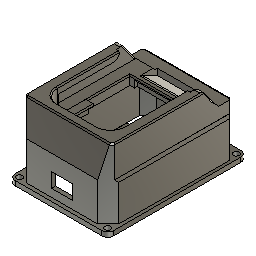
Makita_DIY_Akkulampe (Autodesk Fusion 360 design; units mm, degrees)
Autodesk Fusion 360 part; units mm, degrees
note: some values were not read from the file. Chosen so that the rebuilt part matches the saved one: a side; which face or edge a step refers to; which pieces of a blend or face edit are solid. Set by a fixed rule: which sketch regions a step uses.
sketch "Sketch1" plane through (0, 0, 0) normal (0, 0, 1) x (1, 0, 0)
  line L0 (42.5, 60) -> (-42.5, 60)
  line L1 (-42.5, 60) -> (-42.5, -60)
  line L2 (-42.5, -60) -> (42.5, -60)
  line L3 (42.5, -60) -> (42.5, 60)
  line L4 (42.5, 60) -> (-42.5, -60) construction
  line L5 (-42.5, 60) -> (42.5, -60) construction
  line L6 (-38, 55.5) -> (38, 55.5) construction
  line L7 (38, 55.5) -> (38, -55.5) construction
  line L8 (38, -55.5) -> (-38, -55.5) construction
  line L9 (-38, -55.5) -> (-38, 55.5) construction
  line L10 (-38, 55.5) -> (38, -55.5) construction
  line L11 (38, 55.5) -> (-38, -55.5) construction
  circle A0 centre (-38, -55.5) radius 2.5
  circle A1 centre (38, -55.5) radius 2.5
  circle A2 centre (38, 55.5) radius 2.5
  circle A3 centre (-38, 55.5) radius 2.5
  line L12 (29.2374, -53.4062) -> (-29.365, -53.4062)
  line L13 (-29.365, 53.5938) -> (29.4929, 53.5938)
  line L14 (36.3085, -53.4062) -> (-36.436, 53.5938) construction
  line L15 (-36.436, -53.4062) -> (36.564, 53.5938) construction
  line L16 (-36.436, -46.3352) -> (-29.365, -53.4062)
  line L17 (29.2374, -53.4062) -> (36.3085, -46.3352)
  line L18 (29.4929, 53.5938) -> (36.564, 46.5227)
  line L19 (-36.436, 46.5227) -> (-29.365, 53.5938)
  line L20 (-32.9005, 50.0582) -> (-36.436, 53.5938) construction
  line L21 (33.0284, 50.0582) -> (36.564, 53.5938) construction
  line L22 (32.773, -49.8707) -> (36.3085, -53.4062) construction
  line L23 (-36.436, -53.4062) -> (-32.9005, -49.8707) construction
  line L24 (-36.436, -46.3352) -> (-36.436, 46.5227)
  line L25 (36.564, 46.5227) -> (36.3085, -46.3352)
  line L26 (-29.862, 54.7938) -> (29.99, 54.7938)
  line L27 (29.99, 54.7938) -> (37.7653, 47.0184)
  line L28 (37.7653, 47.0184) -> (37.5071, -46.8336)
  line L29 (29.7345, -54.6062) -> (37.5071, -46.8336)
  line L30 (29.7345, -54.6062) -> (-29.862, -54.6062)
  line L31 (-37.636, -46.8322) -> (-29.862, -54.6062)
  line L32 (-37.636, -46.8322) -> (-37.636, 47.0198)
  line L33 (-37.636, 47.0198) -> (-29.862, 54.7938)
  line L34 (-30.8147, 57.0938) -> (30.9427, 57.0938)
  line L35 (30.9427, 57.0938) -> (40.068, 47.9685)
  line L36 (40.068, 47.9685) -> (39.8045, -47.7889)
  line L37 (30.6872, -56.9062) -> (39.8045, -47.7889)
  line L38 (30.6872, -56.9062) -> (-30.8147, -56.9062)
  line L39 (-39.936, -47.7849) -> (-30.8147, -56.9062)
  line L40 (-39.936, -47.7849) -> (-39.936, 47.9725)
  line L41 (-39.936, 47.9725) -> (-30.8147, 57.0938)
  line L42 (31.5, -44.5) -> (-31.5, 44.5) construction
  line L43 (-31.5, -44.5) -> (31.5, 44.5) construction
  line L44 (-28.5365, 51.5938) -> (28.6645, 51.5938)
  line L45 (28.6645, 51.5938) -> (34.5617, 45.6966)
  line L46 (34.5617, 45.6966) -> (34.3108, -45.5044)
  line L47 (28.409, -51.4062) -> (34.3108, -45.5044)
  line L48 (28.409, -51.4062) -> (-28.5365, -51.4062)
  line L49 (-34.436, -45.5067) -> (-28.5365, -51.4062)
  line L50 (-34.436, -45.5067) -> (-34.436, 45.6943)
  line L51 (-34.436, 45.6943) -> (-28.5365, 51.5938)
  dimension "d1" = 85
  dimension "d2" = 120
  dimension "d3" = 76
  dimension "d4" = 111
  dimension "d5" = 5
  dimension "d6" = 73
  dimension "d7" = 107
  dimension "d9" = 10
  dimension "d10" = 1.2
  dimension "d11" = 3.5
  dimension "d20" = 89
  dimension "d21" = 63
  dimension "d33" = 2
  constraint perpendicular L0 L1
  constraint parallel L0 L2
  constraint parallel L1 L3
  constraint horizontal L0
  constraint perpendicular L6 L7
  constraint parallel L6 L8
  constraint parallel L7 L9
  constraint horizontal L6
  constraint coincident L8.end L9.start
  constraint coincident L7.end L8.start
  constraint coincident L6.end L7.start
  constraint coincident L6.start L9.end
  constraint equal A0 A1
  constraint equal A0 A3
  constraint equal A2 A3
  constraint perpendicular L12 L24
  constraint parallel L12 L13
  constraint horizontal L12
  constraint midpoint L19 L20.start
  constraint perpendicular L19 L20
  constraint midpoint L18 L21.start
  constraint perpendicular L18 L21
  constraint midpoint L17 L22.start
  constraint perpendicular L17 L22
  constraint midpoint L16 L23.end
  constraint perpendicular L16 L23
  constraint equal L22 L23
  constraint equal L20 L23
  constraint equal L20 L21
  constraint horizontal L15.start L12.end
  constraint vertical L15.start L16.start
  constraint vertical L14.start L17.end
  constraint horizontal L14.start L12.start
  constraint horizontal L15.end L13.end
  constraint vertical L15.end L18.end
  constraint vertical L14.end L19.start
  constraint horizontal L14.end L13.start
  measures "d1" distance of L1.end L2.end
  measures "d2" distance of L0.end L1.end
  measures "d3" distance of L7.end L8.end
  measures "d4" distance of L6.end L7.end
  measures "d5" diameter of A2
  measures "d6" distance of L14.end L15.end
  measures "d7" distance of L15.start L14.end
  measures "d9" distance of L13.end L18.end
  measures "d20" distance of L42.start L43.end
  measures "d21" distance of L42.start L43.start
extrude "Extrude5" add sketch "Sketch1" against normal blind 2 contours L0 L1 L2 L3 | L12 L13 L16 L17 L18 L19 L24 L25 | L26 L27 L28 L29 L30 L31 L32 L33 | L44 L45 L46 L47 L48 L49 L50 L51 makes body 1 at (10.2291, -58.9687, 0) makes body 2 at (12.5455, 15.7349, 0)
extrude "Extrude6" add sketch "Sketch1" along normal blind 2 contours L0 L1 L2 L3 | L12 L13 L16 L17 L18 L19 L24 L25 | L26 L27 L28 L29 L30 L31 L32 L33 | L34 L35 L36 L37 L38 L39 L40 L41 | L44 L45 L46 L47 L48 L49 L50 L51 bodies 1 2
sketch "Sketch1 (2)" plane through (0, 0, 0) normal (0, 0, 1) x (1, 0, 0) in component "Contacts"
  line L0 (0, 21.9) -> (8.9, 21.9)
  line L1 (8.9, 21.9) -> (8.9, -21.9)
  line L2 (8.9, -21.9) -> (0, -21.9)
  line L3 (8.9, 14.4) -> (24.3, 14.4)
  line L4 (24.3, 14.4) -> (24.3, -14.4)
  line L5 (24.3, -14.4) -> (8.9, -14.4)
  line L6 (0, 21.9) -> (-30.1, 21.9)
  line L7 (-30.1, 21.9) -> (-30.1, -21.9)
  line L8 (-30.1, -21.9) -> (0, -21.9)
  line L9 (0, -21.9) -> (0, 21.9)
  line L10 (8.9, 14.4) -> (26.7, 14.4)
  line L11 (26.7, 14.4) -> (26.7, 18.8)
  line L12 (26.7, 18.8) -> (8.9, 18.8)
  line L13 (8.9, 18.8) -> (8.9, 14.4)
  line L14 (8.9, -14.4) -> (26.7, -14.4)
  line L15 (26.7, -14.4) -> (26.7, -18.8)
  line L16 (26.7, -18.8) -> (8.9, -18.8)
  line L17 (8.9, -18.8) -> (8.9, -14.4)
  line L18 (-30.1, 17.6) -> (0, 17.6)
  line L19 (0, -17.6) -> (-30.1, -17.6)
  line L20 (-30.1, -17.6) -> (-30.1, 17.6)
  line L21 (-30.1, 17.6) -> (-32.5, 17.6)
  line L22 (-32.5, 17.6) -> (-32.5, -17.6)
  line L23 (-32.5, -17.6) -> (-30.1, -17.6)
  line L24 (-30.1, -17.6) -> (-30.1, 17.6)
  line L25 (0, 0) -> (41.4806, 0) construction
  point P0 (24.3, 0)
  dimension "d34" = 28.8
  dimension "d35" = 15.4
  dimension "d36" = 17.8
  dimension "d39" = 54.4
  dimension "d40" = 24.3
  dimension "d41" = 4.3
  dimension "d42" = 2.4
  dimension "d43" = 35.2
  dimension "d44" = 37.6
  constraint horizontal L0
  constraint vertical L1
  constraint horizontal L2
  constraint horizontal L3
  constraint vertical L4
  constraint horizontal L5
  constraint coincident L1 L3.start
  constraint horizontal L6
  constraint vertical L7
  constraint horizontal L8
  constraint vertical L9
  constraint horizontal L10
  constraint vertical L11
  constraint horizontal L12
  constraint vertical L13
  constraint horizontal L14
  constraint vertical L15
  constraint horizontal L16
  constraint vertical L17
  constraint collinear L11 L15
  constraint equal L11 L15
  constraint horizontal L18
  constraint horizontal L19
  constraint vertical L20
  constraint coincident L7 L18.start
  constraint midpoint L7 L20
  constraint horizontal L21
  constraint vertical L22
  constraint horizontal L23
  constraint vertical L24
  constraint coincident L19.end L20.start
  constraint midpoint L25.start L9
  constraint coincident L1 L5.end
  constraint coincident L25.start origin
  constraint coincident L4 P0
  constraint midpoint L4 P0
  constraint coincident L25 P0
  constraint coincident L9 L18.end
  constraint coincident L9 L19.start
  constraint coincident L2.end L8.end
  constraint horizontal L25
  measures "d34" distance of L3.start L5.end
  measures "d35" distance of L3.start L3.end
  measures "d36" distance of L11.end L12.end
  measures "d39" distance of L4 L7
  measures "d40" horizontal distance of L0.start L3.end
  measures "d41" distance of L6.end L18.start
  measures "d42" distance of L22.end L19.end
  measures "d43" distance of L18.start L19.end
  measures "d44" distance of L11.end L15.end
extrude "Extrude1" add sketch "Sketch1 (2)" along normal blind 2 separate body contours L7 L9 L18 L19 L20 L24 | L1 L3 L10 L11 L12 L13 | L1 L5 L14 L15 L16 L17 makes body 3 at (-20.0667, 5.8667, 0) makes body 4 at (14.8333, -17.3333, 0) makes body 5 at (14.8333, 15.8667, 0) in component "Contacts"
extrude "Extrude2" add sketch "Sketch1 (2)" along normal blind 13.5 contours L0 L1 L2 L9 L13 L17 | L1 L3 L4 L5 L10 L14 bodies 3 4 5 in component "Contacts"
extrude "Extrude3" add sketch "Sketch1 (2)" along normal blind 4.5 contours L6 L7 L9 L18 | L7 L8 L9 L19 bodies 3 in component "Contacts"
extrude "Extrude4" add sketch "Sketch1 (2)" against normal blind 2 separate body contours L7 L20 L21 L22 L23 L24 makes body 6 in component "Contacts"
extrude "Extrude5'" add 1 faces at (-30.1, 5.8667, -0.6667) along direction (1, 0, 0) blind 2 on bodies 6 bodies 6 3 in component "Contacts"
sketch "Sketch2" plane through (0, 0, 4.5) normal (0, 0, 1) x (-1, 0, 0) in component "Contacts"
  line L0 (30.1, -17.6) -> (0, -17.6)
  line L1 (0, -17.6) -> (0, -21.9)
  line L2 (0, -21.9) -> (30.1, -21.9)
  line L3 (30.1, -21.9) -> (30.1, -17.6)
  line L4 (25.4, -20) -> (0, -20)
  line L5 (0, -20) -> (0, -19)
  line L6 (0, -19) -> (25.4, -19)
  line L7 (25.4, -19) -> (25.4, -20)
  line L8 (25.4, 19) -> (0, 19)
  line L9 (0, 19) -> (0, 20)
  line L10 (0, 20) -> (25.4, 20)
  line L11 (25.4, 20) -> (25.4, 19)
  line L12 (0, 0) -> (12.7, 0) construction
  line L13 (12.7, 0) -> (12.7, -19) construction
  line L14 (12.7, 0) -> (12.7, 19) construction
  dimension "d55" = 40
  dimension "d56" = 1
  dimension "d57" = 25.4
  constraint horizontal L4
  constraint vertical L5
  constraint horizontal L6
  constraint vertical L7
  constraint coincident L1 L5.end
  constraint horizontal L8
  constraint vertical L9
  constraint horizontal L10
  constraint vertical L11
  constraint collinear L7 L11
  constraint coincident L12.start origin
  constraint parallel L6 L12
  constraint midpoint L6 L13.end
  constraint perpendicular L6 L13
  constraint midpoint L8 L14.end
  constraint perpendicular L8 L14
  constraint equal L13 L14
  constraint equal L7 L11
  measures "d55" distance of L4.start L10.end
  measures "d56" distance of L4.start L6.end
  measures "d57" distance of L5.end L6.end
extrude "Extrude6'" add sketch "Sketch2" along normal blind 8.3 contours L1 L4 L5 L6 L7 | L8 L9 L10 L11 bodies 6 in component "Contacts"
extrude "Extrude7" add sketch "Sketch1" along normal blind 35 contours L26 L27 L28 L29 L30 L31 L32 L33 | L34 L35 L36 L37 L38 L39 L40 L41 bodies 1
extrude "Extrude8" cut 1 faces at (12.1455, 15.5701, 2) along direction (0, 0, -1) blind 26 on bodies 1 bodies 1
sketch "Sketch2 (2)" plane through (0, 0, 35) normal (0, 0, 1) x (-1, 0, 0)
  line L0 (29.365, 53.4062) -> (36.436, 46.3352)
  line L1 (36.436, 46.3352) -> (36.436, -46.5227)
  line L2 (36.436, -46.5227) -> (29.365, -53.5938)
  line L3 (29.365, -53.5938) -> (-29.4929, -53.5938)
  line L4 (-29.4929, -53.5938) -> (-36.564, -46.5227)
  line L5 (-36.564, -46.5227) -> (-36.3085, 46.3352)
  line L6 (-36.3085, 46.3352) -> (-29.2374, 53.4062)
  line L7 (-29.2374, 53.4062) -> (29.365, 53.4062)
  line L8 (39.936, 47.7849) -> (30.8147, 56.9062)
  line L9 (30.8147, 56.9062) -> (-30.6872, 56.9062)
  line L10 (-30.6872, 56.9062) -> (-39.8045, 47.7889)
  line L11 (-39.8045, 47.7889) -> (-40.068, -47.9685)
  line L12 (-40.068, -47.9685) -> (-30.9427, -57.0938)
  line L13 (-30.9427, -57.0938) -> (30.8147, -57.0938)
  line L14 (30.8147, -57.0938) -> (39.936, -47.9725)
  line L15 (39.936, -47.9725) -> (39.936, 47.7849)
  line L16 (-38, -51.65) -> (38, -51.65)
  line L17 (38, -51.65) -> (38, 51.65)
  line L18 (38, 51.65) -> (-38, 51.65)
  line L19 (-38, 51.65) -> (-38, -51.65)
  line L20 (-38, -51.65) -> (38, 51.65) construction
  line L21 (38, -51.65) -> (-38, 51.65) construction
  line L22 (29, -38.65) -> (29, 32.03)
  line L23 (-29, 32.03) -> (-29, -38.65)
  line L24 (17, 44.03) -> (-17, 44.03)
  arc A0 (29, 32.03) -> (17, 44.03) centre (17, 32.03) ccw
  arc A1 (-17, 44.03) -> (-29, 32.03) centre (-17, 32.03) ccw
  line L25 (38, -38.65) -> (-38, -38.65)
  line L26 (-17, -28.3) -> (17, -28.3)
  line L27 (17, -28.3) -> (17, -42.3)
  line L28 (17, -42.3) -> (-17, -42.3)
  line L29 (-17, -42.3) -> (-17, -28.3)
  line L30 (-17, -28.3) -> (17, -42.3) construction
  line L31 (17, -28.3) -> (-17, -42.3) construction
  line L32 (0, -35.3) -> (0, -51.65) construction
  line L33 (-22, -23.65) -> (22, -23.65)
  line L34 (22, -23.65) -> (22, 15.55)
  line L35 (22, 15.55) -> (-22, 15.55)
  line L36 (-22, 15.55) -> (-22, -23.65)
  line L37 (-22, -23.65) -> (22, 15.55) construction
  line L38 (22, -23.65) -> (-22, 15.55) construction
  line L39 (14.5, 15.55) -> (-14.5, 15.55)
  line L40 (-14.5, 15.55) -> (-14.5, 30.65)
  line L41 (-14.5, 30.65) -> (14.5, 30.65)
  line L42 (14.5, 30.65) -> (14.5, 15.55)
  point P0 (0, -35.3)
  point P1 (0, -4.05)
  dimension "d64" = 76
  dimension "d65" = 103.3
  dimension "d66" = 7.62
  dimension "d67" = 9
  dimension "d68" = 9
  dimension "d69" = 12
  dimension "d70" = 12
  dimension "d71" = 13
  dimension "d72" = 9.35
  dimension "d73" = 34
  dimension "d74" = 14
  dimension "d76" = 28
  dimension "d77" = 44
  dimension "d78" = 39.2
  dimension "d79" = 54.3
  dimension "d80" = 29
  constraint perpendicular L16 L17
  constraint parallel L16 L18
  constraint parallel L17 L19
  constraint horizontal L16
  constraint coincident L20 origin
  constraint coincident L21 origin
  constraint vertical L22
  constraint parallel L22 L23
  constraint perpendicular L22 L24
  constraint tangent L22 A0
  constraint tangent L24 A0
  constraint tangent L24 A1
  constraint tangent L23 A1
  constraint coincident L17 L25.start
  constraint coincident L19 L25.end
  constraint perpendicular L19 L25
  constraint perpendicular L26 L27
  constraint parallel L26 L28
  constraint parallel L27 L29
  constraint horizontal L26
  constraint coincident L30 P0
  constraint coincident L31 P0
  constraint midpoint L31 P0
  constraint coincident P0 L32.start
  constraint midpoint L16 L32.end
  constraint vertical L32
  constraint horizontal L22.start L23.end
  constraint coincident L22.start L25
  constraint perpendicular L33 L34
  constraint parallel L33 L35
  constraint parallel L34 L36
  constraint horizontal L33
  constraint coincident L37 P1
  constraint coincident L38 P1
  constraint vertical origin P1
  constraint horizontal L39
  constraint vertical L40
  constraint horizontal L41
  constraint vertical L42
  constraint coincident L35 L39.start
  constraint midpoint L35 L39
  measures "d64" distance of L16.start L16.end
  measures "d65" distance of L16.start L18.end
  measures "d66" distance of L18 L24
  measures "d67" distance of L17 L22
  measures "d68" distance of L19 L23
  measures "d69" radius of A0
  measures "d70" radius of A1
  measures "d71" distance of L16 L25
  measures "d72" distance of L16 L28
  measures "d73" distance of L27.end L28.end
  measures "d74" distance of L26.start L28.end
  measures "d76" distance of L16 L33
  measures "d77" distance of L34.end L35.end
  measures "d78" distance of L33.end L34.end
  measures "d79" distance of L33 L40.end
  measures "d80" distance of L40.end L41.end
extrude "Extrude9" add sketch "Sketch2 (2)" along normal blind 27 contours L0 L1 L8 L17 L18 L25 | L0 L1 L5 L6 L18 L22 L23 L24 A0 A1 L25 | L5 L6 L10 L18 L19 L25 bodies 1
extrude "Extrude10" add sketch "Sketch2 (2)" along normal blind 11.8 contours L22 L23 L24 A0 A1 L25 L26 L27 L29 bodies 1
extrude "Extrude11" add sketch "Sketch2 (2)" along normal blind 10.1 separate body contours L1 L2 L14 L16 L17 L25 | L1 L2 L4 L5 L16 L25 L27 L28 L29 | L4 L5 L12 L16 L19 L25 makes body 7
sketch "Sketch3" plane through (0, 0, 0) normal (1, 0, 0) x (0, 1, 0)
  line L0 (38.65, 46.8) -> (-32.03, 46.8)
  line L1 (-51.65, 35) -> (-51.65, 62)
  line L2 (-51.65, 62) -> (-51.65, 35)
  line L3 (-35.598, 46.8) -> (31.1855, 46.8)
  line L4 (31.1855, 46.8) -> (31.1855, 56.4)
  line L5 (31.1855, 56.4) -> (-31.35, 56.4)
  line L6 (31.1855, 56.4) -> (21.65, 56.4)
  line L7 (21.65, 56.4) -> (21.65, 62)
  line L8 (21.65, 62) -> (31.1855, 62)
  line L9 (31.1855, 62) -> (31.1855, 56.4)
  line L10 (-31.35, 56.4) -> (-31.35, 46.8)
  line L11 (38.65, 62) -> (-32.03, 62)
  line L12 (38.65, 46.8) -> (27.65, 62)
  line L13 (38.65, 62) -> (38.65, 46.8)
  line L14 (42.3, 35) -> (42.3, 45.1)
  line L15 (42.3, 45.1) -> (42.3, 35)
  line L16 (28.3, 35) -> (28.3, 46.8)
  line L17 (28.3, 46.8) -> (28.3, 35)
  line L18 (42.3, 35) -> (28.3, 35)
  line L19 (28.3, 46.8) -> (42.3, 39.6)
  dimension "d87" = 20.3
  dimension "d88" = 73.3
  dimension "d89" = 5.6
  dimension "d90" = 79.3
  dimension "d95" = 5.5
  constraint horizontal L3
  constraint vertical L4
  constraint horizontal L5
  constraint horizontal L6
  constraint vertical L7
  constraint horizontal L8
  constraint vertical L9
  constraint perpendicular L0 L10
  constraint horizontal L8.end L11.start
  constraint coincident L3 L10.end
  constraint coincident L0.end L3
  constraint coincident L0.start L12.start
  constraint coincident L11 L12.end
  constraint coincident L11.start L13.start
  constraint coincident L14.start L15.end
  constraint coincident L16.start L17.end
  constraint coincident L16.end L17.start
  constraint coincident L15 L19.end
  measures "d87" distance of L2 L5.end
  measures "d88" distance of L1.end L7
  measures "d89" vertical distance of L5.end L11.end
  measures "d90" distance of L1.end L12.end
  measures "d95" distance of L14.end L19.end
extrude "Extrude12" cut sketch "Sketch3" along normal up to surface (38 mm away) contours L9 L11 L12 L13 | L8 L9 L11 L12 bodies 1
extrude "Extrude13" cut sketch "Sketch3" along normal up to surface (31.9 mm away) contours L0 L4 L9 L12 | L0 L3 L4 L5 L6 L10 | L5 L6 L7 L8 L9 L11 L12 bodies 1
extrude "Extrude14" add sketch "Sketch3" along normal up to surface (17 mm away) contours L14 L15 L16 L17 L18 L19 bodies 1 7
mirror "Mirror1" about plane through (0, 0, 0) normal (1, 0, 0) of "Extrude12", "Extrude13", "Extrude14"
sketch "Sketch4" plane through (0, 0, 35) normal (0, 0, 1) x (1, 0, 0)
  line L0 (22, 23.65) -> (-22, 23.65)
  line L1 (18, 23.65) -> (-18, 23.65)
  line L2 (-18, 23.65) -> (-18, 26.15)
  line L3 (-18, 26.15) -> (18, 26.15)
  line L4 (18, 26.15) -> (18, 23.65)
  line L5 (0, 0) -> (0, 23.65) construction
  line L6 (-14.5, -15.55) -> (14.5, -15.55)
  line L7 (-18.9, -15.55) -> (18.9, -15.55)
  line L8 (18.9, -15.55) -> (18.9, -33.05)
  line L9 (18.9, -33.05) -> (-18.9, -33.05)
  line L10 (-18.9, -33.05) -> (-18.9, -15.55)
  line L11 (-22, -15.55) -> (22, -15.55)
  line L12 (14.5, -15.55) -> (14.5, -30.65)
  line L13 (14.5, -30.65) -> (-14.5, -30.65)
  line L14 (-14.5, -30.65) -> (-14.5, -15.55)
  line L15 (-20.9, -13.55) -> (20.9, -13.55)
  line L16 (20.9, -13.55) -> (20.9, -35.05)
  line L17 (20.9, -35.05) -> (-20.9, -35.05)
  line L18 (-20.9, -35.05) -> (-20.9, -13.55)
  line L19 (17, -44.03) -> (-17, -44.03)
  line L20 (-14.5, -30.65) -> (-14.5, -33.05)
  line L21 (14.5, -30.65) -> (14.5, -33.05)
  line L22 (-14.5, -33.05) -> (-14.5, -44.03)
  line L23 (14.5, -33.05) -> (14.5, -44.03)
  dimension "d99" = 36
  dimension "d100" = 2.5
  dimension "d103" = 37.8
  dimension "d104" = 17.5
  dimension "d110" = -2
  constraint horizontal L1
  constraint vertical L2
  constraint horizontal L3
  constraint vertical L4
  constraint coincident L0 L1.start
  constraint coincident L5.start origin
  constraint midpoint L1 L5.end
  constraint vertical L5
  constraint horizontal L7
  constraint vertical L8
  constraint horizontal L9
  constraint vertical L10
  constraint midpoint L7 L11
  constraint coincident L13.end L14.start
  constraint coincident L9 L20.end
  constraint perpendicular L9 L20
  constraint coincident L12.end L13.start
  constraint coincident L9 L21.end
  constraint perpendicular L9 L21
  constraint coincident L19 L22.end
  constraint perpendicular L19 L22
  constraint coincident L19 L23.end
  constraint perpendicular L19 L23
  measures "d99" distance of L2.end L3.end
  measures "d100" distance of L1.end L2.end
  measures "d103" distance of L8.end L9.end
  measures "d104" distance of L7.end L8.end
extrude "Extrude15" cut sketch "Sketch4" along normal up to surface (9.8 mm away) contours L0 L1 L2 L3 L4 bodies 1
extrude "Extrude16" cut sketch "Sketch4" along normal up to surface (11.8 mm away) contours L7 L9 L10 L11 L14 L20 | L6 L7 L11 L12 L13 L14 | L7 L8 L9 L11 L12 L21 | L9 L13 L20 L21 | L9 L17 L22 L23 | L17 L19 L22 L23 bodies 1
extrude "Extrude17" add sketch "Sketch4" along normal blind 2 from surface at 11.8 contours L7 L9 L10 L11 L14 L20 | L7 L8 L9 L11 L12 L21 | L9 L10 L11 L17 L18 L22 | L8 L9 L11 L16 L17 L23 bodies 1
sketch "Sketch5" plane through (0, 0, 0) normal (1, 0, 0) x (0, 1, 0)
  line L0 (-51.65, 35) -> (-51.65, 62)
  line L1 (-51.65, 62) -> (-51.65, 35)
  line L2 (-51.65, 35) -> (-53.4062, 35)
  line L3 (-53.4062, 35) -> (-51.65, 35)
  line L4 (-51.65, 35) -> (-56.9062, 35)
  line L5 (-56.9062, 35) -> (-51.65, 35)
  line L6 (-56.9062, 35) -> (-51.65, 62)
  line L7 (51.65, 35) -> (53.5938, 35)
  line L8 (53.5938, 35) -> (51.65, 35)
  line L9 (51.65, 35) -> (57.0938, 35)
  line L10 (57.0938, 35) -> (51.65, 35)
  line L11 (51.65, 35) -> (51.65, 45.1)
  line L12 (51.65, 45.1) -> (51.65, 35)
  line L13 (57.0938, 35) -> (51.65, 45.1)
  constraint coincident L4.end L5.start
  constraint coincident L0.end L1.start
  constraint coincident L9.end L10.start
  constraint coincident L11.end L12.start
extrude "Extrude18" add sketch "Sketch5" along normal mid plane 74 bodies 1
extrude "Extrude19" cut 4 faces at (34.5435, -55.1541, 35) (34.7764, 55.2792, 35) (-34.6911, 55.2792, 35) (-34.6285, -55.1541, 35) along direction (0, 0, 1) blind 37 on bodies 1 bodies 1
chamfer "Chamfer4" distance 1.7 angle 45 2 edges at (27.5, 38.65, 45.1) (-27.5, 38.65, 45.1) on bodies 1
fillet "Fillet2" radius 1 2 edges at (-20.9, -25.3, 46.8) (20.9, -25.3, 46.8) on bodies 1
fillet "Fillet3" radius 5 8 edges at (34.95, 27.65, 62) (-34.95, 27.65, 62) (30.45, 21.65, 56.4) (-30.45, 21.65, 56.4) (42.5, 60, 0) (-42.5, 60, 0) (42.5, -60, 0) (-42.5, -60, 0) on bodies 1
chamfer "Chamfer5" distance 1 angle 45 21 edges at (-38, -11.0355, 62) (-37.0355, -50.6855, 62) (-0.0638, -51.65, 62) (38, -10.9717, 62) (36.9717, -50.6217, 62) (0, 23.65, 46.8) (22, 4.05, 46.8) (14.5, -39.54, 46.8) (-14.5, -39.54, 46.8) (-22, 4.05, 46.8) (0.064, 51.65, 45.1) (29, -5.19, 62) (25.4853, -40.5153, 62) (0, -44.03, 62) (-25.4853, -40.5153, 62) (-29, -5.19, 62) (-38, 33.15, 54.4) (-31.9, 33.15, 54.4) (31.9, 33.15, 54.4) (38, 33.15, 54.4) (0, 28.3, 46.8) on bodies 1
chamfer "Chamfer6" distance 5 angle 45 8 edges at (0.064, 53.5938, 35) (33.0284, 50.0582, 35) (36.4362, 0.0938, 35) (-36.436, 0.0938, 35) (-32.9005, 50.0582, 35) (-0.0638, -53.4062, 35) (-32.9005, -49.8707, 35) (32.773, -49.8707, 35) on bodies 1
chamfer "Chamfer7" distance 4 angle 45 16 edges at (22, 4.05, 35) (20, 23.65, 35) (0, 26.15, 35) (18, 24.9, 35) (20.45, -15.55, 35) (18.9, -24.3, 35) (16.7, -33.05, 35) (14.5, -38.54, 35) (0, -44.03, 35) (-14.5, -38.54, 35) (-18.9, -24.3, 35) (-22, 4.05, 35) (-18, 24.9, 35) (-20, 23.65, 35) (-20.45, -15.55, 35) (-16.7, -33.05, 35) on bodies 1
sketch "Sketch6" plane through (0, -56.9062, 0) normal (0, -1, 0) x (1, 0, 0)
  line L0 (-30.8147, 2) -> (30.6872, 2)
  line L1 (30.6872, 2) -> (30.6872, 35)
  line L2 (30.6872, 35) -> (-30.8147, 35)
  line L3 (-30.8147, 35) -> (-30.8147, 2)
  line L4 (9.25, 21.25) -> (-9.25, 21.25)
  line L5 (-9.25, 21.25) -> (-9.25, 8.75)
  line L6 (-9.25, 8.75) -> (9.25, 8.75)
  line L7 (9.25, 8.75) -> (9.25, 21.25)
  line L8 (9.25, 21.25) -> (-9.25, 8.75) construction
  line L9 (-9.25, 21.25) -> (9.25, 8.75) construction
  point P0 (0, 15)
  dimension "d122" = 18.5
  dimension "d123" = 12.5
  dimension "d124" = 15
  constraint perpendicular L4 L5
  constraint parallel L4 L6
  constraint parallel L5 L7
  constraint horizontal L4
  constraint coincident L8 P0
  constraint coincident L9 P0
  constraint vertical origin P0
  measures "d122" distance of L4.start L4.end
  measures "d123" distance of L4.start L6.end
  measures "d124" distance of origin P0
extrude "Extrude20" cut sketch "Sketch6" against normal up to surface (3.5 mm away) contours L4 L5 L6 L7 bodies 1
chamfer "Chamfer8" distance 1.9 angle 45 2 edges at (-39.936, 0.0938, 35) (39.9362, 0.0898, 35) on bodies 1
component "Contacts" placed x (1, 0, 0) y (0, 1, 0) z (0, 0, 1) at (0, 0, 0)
